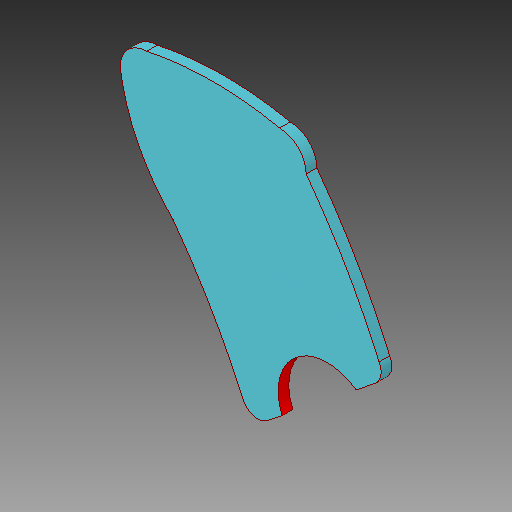
# Autodesk Inventor part: brazocuadrado
Saved by Autodesk Inventor 2019 (Build 230136000, 136)
## iProperties
Part Number: brazocuadrado
Material: Genérico
Document SubType Name: Chapa
Designer: Kevin
Density: 1 g/cm^3
Sheet Metal Rule: Por defecto_mm
Appearance: Valor por defecto
Author: Kevin
Autodesk Inventor part; units mm, degrees
ref_plane "YZ Plane" through (0, 0, 0) normal (1, 0, 0) x (0, 1, 0)
ref_plane "Plano de trabajo14" through (0, 0, 40) normal (0, 0, 1) x (1, 0, 0)
ref_plane "Plano de trabajo15" through (0, 0, 40) normal (0, 0, -1) x (-1, 0, 0)
sketch "Boceto24" plane through (0, 0, 40) normal (0, 0, -1) x (-1, 0, 0)
  arc A0 (0, 95) -> (-5, 100) centre (-5, 95) ccw
  arc A1 (-30, 100) -> (-35, 95) centre (-30, 95) ccw
  arc A2 (-5, 100) -> (-30, 100) centre (-17.5, 41.3165) ccw
  arc A3 (-10, 75) -> (0, 95) centre (-34.6648, 99.8324) ccw
  line L0 (-47.9872, 67.409) -> (-27.7264, 51.2004)
  arc A4 (-27.7264, 51.2004) -> (-23.2542, 52.043) centre (-25.8523, 53.543) ccw
  arc A5 (-48.7112, 71.2516) -> (-47.9872, 67.409) centre (-46.1131, 69.7516) ccw
  arc A6 (-35, 95) -> (-48.7112, 71.2516) centre (61.3869, 23.5187) ccw
  arc A7 (-10, 75) -> (-23.2542, 52.043) centre (86.6601, 3.8886) ccw
  point P0 (0, 0)
  point P1 (0, 100)
  point P2 (-35, 100)
  point P3 (-25, 49.0192)
  point P4 (-50, 69.0192)
  constraints: 16 point on circle, 8 centre point, 2 end point, 2 point on line
extrude "Extrusión16" add sketch "Boceto24" along normal blind 2
sketch "Boceto34" plane through (0, 0, 40) normal (0, 0, 1) x (1, 0, 0)
  line L0 (30.8918, 53.7327) -> (44.3961, 64.5361)
  line L1 (37.8568, 59.3047) -> (40.3278, 59.3047) construction
  line L2 (30.466, 53.3921) -> (44.3961, 64.5361)
  line L3 (30.466, 53.3921) -> (37.431, 58.9641)
  line L4 (37.431, 58.9641) -> (39.902, 58.9641) construction
  arc A0 (44.3961, 64.5361) -> (30.466, 53.3921) centre (38.9746, 57.0346) ccw
  point P0 (0, 0)
  constraints: 10 end point, 3 point on circle, 2 horizontal, 1 centre point, 1 point on line
extrude "Extrusión26" cut sketch "Boceto34" against normal blind 10
equation "\"Radio_pliegue\" = Grosor"
equation "\"Anchura_desahogo_plegado\" = Grosor"
equation "\"Profundidad_desahogo_plegado\" = 0.5 * Grosor"
equation "\"Tamaño_destalonado\" = 4 * Grosor"
equation "\"Remanente_mínimo\" = 2 * Grosor"
equation "\"Radiodetransición\" = Radio_pliegue"
equation "\"Tamaño_de_radio_de_Jacobi\" = Radio_pliegue"
equation "\"TamañoSeparación\" = Grosor"
equation "\"Grosor\" = 0.5"
